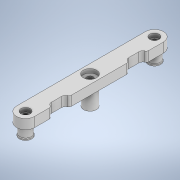
# Autodesk Inventor part: ActuatorLink
Saved by Autodesk Inventor 2022.6 (Build 266554000, 554)
## iProperties
Created: 2024-10-23
Part Number: ActuatorLink
Material: Generic
Document SubType Name: Modeling
Designer: Zhong
Density: 1 g/cm^3
Appearance: Default
Author: Zhong
Autodesk Inventor part; units mm, degrees
ref_plane "YZ Plane" through (0, 0, 0) normal (1, 0, 0) x (0, 1, 0)
ref_plane "XZ Plane" through (0, 0, 0) normal (0, 1, 0) x (-1, 0, 0)
ref_plane "XY Plane" through (0, 0, 0) normal (0, 0, 1) x (1, 0, 0)
sketch "Sketch1" plane through (0, 0, 0) normal (0, 1, 0) x (-1, 0, 0)
  line L0 (0, 25) -> (0, -25) construction
  line L1 (-3.5, 25) -> (-3.5, -25)
  line L2 (3.5, -25) -> (3.5, 25)
  arc A0 (3.5, 25) -> (-3.5, 25) centre (0, 25) ccw
  arc A1 (-3.5, -25) -> (3.5, -25) centre (0, -25) ccw
  point P0 (0, 0)
  point P1 (0, 0)
  dimension "d0" = 50
  dimension "d1" = 7
  constraints: 8 end point, 4 point on circle, 4 tangent, 2 centre point, 1 coincident, 1 midpoint, 1 parallel, 1 vertical
  measures "d0" distance of L0.start L0.end
  measures "d1" diameter of A1
extrude "Extrusion1" add sketch "Sketch1" along normal blind 3.75
sketch "Sketch2" plane through (0, 3.75, 0) normal (0, 1, 0) x (1, 0, 0)
  arc A0 (3.5, 25) -> (-3.5, 25) centre (0, 25) ccw projected
  line L0 (-3.5, 25) -> (-3.5, -25) projected
  arc A1 (-3.5, -25) -> (3.5, -25) centre (0, -25) ccw projected
  line L1 (3.5, -25) -> (3.5, 25) projected
  circle A2 centre (0, 25) radius 1.5
  circle A3 centre (0, -25) radius 1.5
  arc A4 (-3.5, -25) -> (3.5, -25) centre (0, -25) ccw projected
  point P0 (0, 0)
  dimension "d38" = 3
  dimension "d39" = 3
  constraints: 4 coincident, 2 centre point
  measures "d38" diameter of A2
  measures "d39" diameter of A3
sketch "Sketch3" plane through (0, 0, 0) normal (0, -1, 0) x (1, 0, 0)
  arc A0 (-3.5, -25) -> (3.5, -25) centre (0, -25) ccw projected
  line L0 (3.5, 25) -> (3.5, -25) projected
  arc A1 (3.5, 25) -> (-3.5, 25) centre (0, 25) ccw projected
  line L1 (-3.5, -25) -> (-3.5, 25) projected
  circle A2 centre (0, 0) radius 2.5
  circle A3 centre (0, 0) radius 1.2
  dimension "d11" = 5
  dimension "d14" = 2.4
  constraints: 2 centre point, 2 coincident
  measures "d11" diameter of A2
  measures "d14" diameter of A3
extrude "Extrusion2" add sketch "Sketch3" along normal blind 7 contours A2 | A3
sketch "Sketch5" plane through (0, -7, 0) normal (0, -1, 0) x (1, 0, 0)
  point P0 (0, 0)
  point P1 (0, 0)
  constraints: 1 coincident
hole "Hole2" at (0, -7, 0) direction (0, 1, 0) diameter 2.4 depth 10 tip angle 118
sketch "Sketch6" plane through (0, 3.75, 0) normal (0, 1, 0) x (1, 0, 0)
  point P0 (0, 0)
  point P1 (0, 0)
  constraints: 1 coincident
hole "Hole3" at (0, 3.75, 0) direction (0, -1, 0) diameter 5.2 depth 1.5
sketch "Sketch8" plane through (0, 0, 0) normal (0, -1, 0) x (1, 0, 0)
  circle A0 centre (0, 0) radius 2.5 projected
  arc A1 (-3.5, -25) -> (3.5, -25) centre (0, -25) ccw projected
  line L0 (3.5, 25) -> (3.5, -25) projected
  arc A2 (3.5, 25) -> (-3.5, 25) centre (0, 25) ccw projected
  line L1 (-3.5, -25) -> (-3.5, 25) projected
  line L2 (3.5, 25) -> (3.5, -25) projected
  line L3 (3.5, -13) -> (3.5, -17) construction
  line L4 (2, -13) -> (2, -17)
  line L5 (5, -17) -> (5, -13)
  arc A3 (5, -13) -> (2, -13) centre (3.5, -13) ccw
  arc A4 (2, -17) -> (5, -17) centre (3.5, -17) ccw
  line L6 (-5.2, 0) -> (6.7, 0) projected
  line L7 (3.5, 13) -> (3.5, 17) construction
  line L8 (2, 13) -> (2, 17)
  line L9 (5, 17) -> (5, 13)
  arc A5 (2, 13) -> (5, 13) centre (3.5, 13) ccw
  arc A6 (5, 17) -> (2, 17) centre (3.5, 17) ccw
  point P0 (3.5, -15)
  point P1 (3.5, -18.5)
  point P2 (3.5, -11.5)
  point P3 (3.5, 15)
  point P4 (3.5, 11.5)
  point P5 (3.5, 18.5)
  dimension "d32" = 4
  dimension "d33" = 3
  dimension "d34" = 15
  constraints: 16 end point, 8 point on circle, 7 symmetric about line, 4 centre point, 4 tangent, 2 point on line, 1 midpoint, 1 parallel, 2 other
  measures "d32" distance of L3.start L3.end
  measures "d33" diameter of A4
  measures "d34" vertical distance of point (0, 0) point (3.5, -15)
extrude "Extrusion4" cut sketch "Sketch8" against normal through all contours A5 L8 A6 L0 | L0 A4 L4 A3
fillet "Fillet1" radius 1 4 edges at (3.5, 1.875, -11.5) (3.5, 1.875, -18.5) (3.5, 1.875, 18.5) (3.5, 1.875, 11.5)
extrude "Extrusion5" [suppressed]
sketch "Sketch9" plane through (0, 9.55, -25) normal (0, 1, 0) x (1, 0, 0)
  circle A0 centre (0, 0) radius 1.5 projected
  circle A1 centre (0, -50) radius 1.5 projected
  circle A2 centre (0, -50) radius 1.5 projected
  circle A3 centre (0, -50) radius 1.85
  circle A4 centre (0, 0) radius 1.5 projected
  circle A5 centre (0, 0) radius 1.85
  point P0 (0, -25)
  dimension "d42" = 3.7
  dimension "d43" = 3.7
  constraints: 2 centre point, 2 coincident
  measures "d42" diameter of A3
  measures "d43" diameter of A5
extrude "Extrusion6" [suppressed]
chamfer "Chamfer1" [suppressed]
fillet "Fillet2" [suppressed]
sketch "Sketch10" plane through (0, 0, 0) normal (0, -1, 0) x (1, 0, 0)
  arc A0 (3.5, 25) -> (-3.5, 25) centre (0, 25) ccw projected
  arc A1 (-3.5, -25) -> (3.5, -25) centre (0, -25) ccw projected
  circle A2 centre (0, 25) radius 2.25
  circle A3 centre (0, -25) radius 2.25
  point P0 (0, 0)
  dimension "d50" = 4.5
  constraints: 2 centre point, 2 coincident, 1 equal radius
  measures "d50" diameter of A2
extrude "Extrusion7" add sketch "Sketch10" along normal blind 4
sketch "Sketch11" plane through (0, -4, 25) normal (0, -1, 0) x (1, 0, 0)
  circle A0 centre (0, 0) radius 2.25 projected
  circle A1 centre (0, -50) radius 2.25 projected
  circle A2 centre (0, 0) radius 2.4
  circle A3 centre (0, -50) radius 2.4
  point P0 (0, -25)
  dimension "d54" = 4.8
  dimension "d70" = 4.5
  constraints: 2 centre point, 2 coincident, 1 equal radius
  measures "d54" diameter of A2
  measures "d70" diameter of A0
extrude "Extrusion8" add sketch "Sketch11" along normal blind 0.4 contours A0 | A1 | A2 | A3
fillet "Fillet3" radius 0.4 2 edges at (-2.25, -4, 25) (-2.25, -4, -25)
fillet "Fillet4" radius 0.8 3 edges at (-2.25, 0, 25) (-2.25, 0, -25) (-2.5, 0, 0)
sketch "Sketch13" plane through (0, 3.75, 0) normal (0, 1, 0) x (1, 0, 0)
  circle A0 centre (0, -25) radius 2.4 projected
  circle A1 centre (0, 25) radius 2.25 projected
  circle A2 centre (0, -25) radius 3.05 projected
  point P0 (0, 0)
  constraints: 2 coincident
hole "Hole4" at (0, 3.75, 25) at (0, 3.75, -25) direction (0, -1, 0) diameter 2.2 end through all counterbore diameter 3.6 counterbore depth 1.5
equation "\"d43\" = d42"
body "Solid1"
